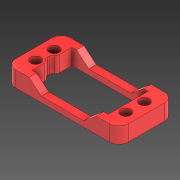
# Autodesk Inventor part: CH_01_0035_servo_mount
Saved by Autodesk Inventor 2022 (Build 260153000, 153)
## iProperties
Created: 2022-04-22
Part Number: CH_01_0035_servo_mount
Material: Acetal Resin, Black
Document SubType Name: Modeling
Designer: Tomasz Krakowski
Density: 1.425 g/cm^3
Appearance: Smooth - Black
Mass: 4.60778 g
Surface Area: 29.6027 cm^2
Volume: 3.23353 cm^3
Author: Tomasz Krakowski
Autodesk Inventor part; units mm, degrees
ref_plane "YZ Plane" through (0, 0, 0) normal (1, 0, 0) x (0, 1, 0)
ref_plane "XZ Plane" through (0, 0, 0) normal (0, 1, 0) x (-1, 0, 0)
ref_plane "XY Plane" through (0, 0, 0) normal (0, 0, 1) x (1, 0, 0)
sketch "Sketch1" plane through (0, 0, 0) normal (0, 1, 0) x (-1, 0, 0)
  line L0 (-20.5, 10.75) -> (20.5, 10.75)
  line L1 (20.5, 10.75) -> (20.5, -10.75)
  line L2 (20.5, -10.75) -> (-20.5, -10.75)
  line L3 (-20.5, -10.75) -> (-20.5, 10.75)
  line L4 (-20.5, 10.75) -> (20.5, -10.75) construction
  line L5 (20.5, 10.75) -> (-20.5, -10.75) construction
  line L6 (-24.25, 5) -> (24.25, 5) construction
  line L7 (24.25, 5) -> (24.25, -5) construction
  line L8 (24.25, -5) -> (-24.25, -5) construction
  line L9 (-24.25, -5) -> (-24.25, 5) construction
  line L10 (-24.25, 5) -> (24.25, -5) construction
  line L11 (24.25, 5) -> (-24.25, -5) construction
  circle A0 centre (24.25, 5) radius 2.75
  circle A1 centre (24.25, -5) radius 2.75
  circle A2 centre (-24.25, 5) radius 2.75
  circle A3 centre (-24.25, -5) radius 2.75
  line L12 (30.25, 9.75) -> (30.25, -9.75)
  line L13 (25.25, -14.75) -> (0, -14.75)
  line L14 (25.25, 14.75) -> (0, 14.75)
  line L15 (0, 14.75) -> (0, 0) construction
  line L16 (0, 0) -> (0, -14.75) construction
  arc A4 (30.25, 9.75) -> (25.25, 14.75) centre (25.25, 9.75) ccw
  arc A5 (25.25, -14.75) -> (30.25, -9.75) centre (25.25, -9.75) ccw
  line L17 (20.5, 2.5) -> (20.5, 2.5)
  line L18 (22.5, 0.5) -> (22.5, -0.5)
  line L19 (20.5, -2.5) -> (20.5, -2.5)
  line L20 (20.5, -2.5) -> (20.5, 2.5)
  line L21 (20.5, 2.5) -> (22.5, -2.5) construction
  line L22 (22.5, 2.5) -> (20.5, -2.5) construction
  line L23 (21.5, 0) -> (0, 0) construction
  line L24 (-30.25, 9.75) -> (-30.25, -9.75)
  line L25 (-25.25, -14.75) -> (0, -14.75)
  line L26 (-25.25, 14.75) -> (0, 14.75)
  arc A6 (-25.25, 14.75) -> (-30.25, 9.75) centre (-25.25, 9.75) ccw
  arc A7 (-30.25, -9.75) -> (-25.25, -14.75) centre (-25.25, -9.75) ccw
  arc A8 (22.5, 0.5) -> (20.5, 2.5) centre (20.5, 0.5) ccw
  arc A9 (20.5, -2.5) -> (22.5, -0.5) centre (20.5, -0.5) ccw
  line L27 (-20.5, 2.5) -> (-20.5, 2.5)
  line L28 (-22.5, 0.5) -> (-22.5, -0.5)
  line L29 (-20.5, -2.5) -> (-20.5, -2.5)
  line L30 (-20.5, -2.5) -> (-20.5, 2.5)
  line L31 (-20.5, 2.5) -> (-22.5, -2.5) construction
  line L32 (-22.5, 2.5) -> (-20.5, -2.5) construction
  arc A10 (-20.5, 2.5) -> (-22.5, 0.5) centre (-20.5, 0.5) ccw
  arc A11 (-22.5, -0.5) -> (-20.5, -2.5) centre (-20.5, -0.5) ccw
  point P0 (20.5, 2.5)
  point P1 (20.5, -2.5)
  point P2 (-21.5, 0)
  point P3 (-20.5, -2.5)
  point P4 (-20.5, 2.5)
  point P5 (20.5, 3.5)
  point P6 (20.5, -3.5)
  point P7 (-20.5, -3.5)
  point P8 (-20.5, 3.5)
  dimension "d0" = 21.5
  dimension "d1" = 41
  dimension "d2" = 5.5
  dimension "d3" = 48.5
  dimension "d4" = 10
  dimension "d5" = 4
  dimension "d6" = 4
  dimension "d7" = 6
  dimension "d8" = 5
  dimension "d9" = 5
  dimension "d10" = 5
  dimension "d11" = 2
  dimension "d12" = 2
  constraints: 66 end point, 17 symmetric about line, 16 point on circle, 12 centre point, 8 midpoint, 8 point on line, 8 tangent, 6 parallel, 5 horizontal, 4 coincident, 4 equal radius, 4 perpendicular, 3 vertical, 1 collinear, 4 other
  measures "d0" distance of L0.end L1.end
  measures "d1" distance between parallel lines of L3 L1
  measures "d2" diameter of A0
  measures "d3" distance between parallel lines of L9 L7
  measures "d4" distance between parallel lines of L8 L6
  measures "d5" distance between parallel lines of L0 L14
  measures "d6" distance between parallel lines of L13 L2
  measures "d7" distance between parallel lines of L7 L12
  measures "d8" radius of A4
  measures "d9" radius of A5
  measures "d10" distance of L22.start L21.end
  measures "d11" distance between parallel lines of L1 L18
  measures "d12" radius of A8
extrude "Extrusion1" add sketch "Sketch1" along normal blind 8.5 contours L3 A11 L28 A10 | L12 A5 L13 L25 A7 L24 A6 L26 L14 A4
sketch "Sketch2" plane through (-25.25, 0, 14.75) normal (0, 0, 1) x (1, 0, 0)
  line L0 (0, 8.5) -> (50.5, 8.5) construction
  line L1 (7.25, 8.5) -> (13.8046, 3)
  line L2 (13.8046, 3) -> (25.25, 3)
  line L3 (25.25, 3) -> (25.25, 8.5)
  line L4 (7.25, 8.5) -> (25.25, 8.5)
  line L5 (43.25, 8.5) -> (36.6954, 3)
  line L6 (36.6954, 3) -> (25.25, 3)
  line L7 (43.25, 8.5) -> (25.25, 8.5)
  point P0 (25.25, 0)
  dimension "d15" = 18
  dimension "d16" = 40
  dimension "d17" = 3
  constraints: 14 end point, 2 symmetric about line, 1 midpoint, 1 parallel, 1 perpendicular, 1 point on line
  measures "d15" distance from line of L3 L1.start
  measures "d16" angle of L0 L1
  measures "d17" distance from line of point (25.25, 0) L2
extrude "Extrusion2" cut sketch "Sketch2" against normal through all
fillet "Fillet1" radius 2 2 edges at (-20.5, 4.25, 2.5) (-20.5, 4.25, -2.5)
equation "\"d6\" = d5"
body "Solid1"
